Autodesk Inventor part; units mm, degrees
(part 2 of 2)
  line L759 (-171.45, -54.625) -> (-171.45, -57.15) construction
  line L760 (-164.45, -59.675) -> (-178.45, -59.675)
  line L761 (-178.45, -59.675) -> (-178.45, -60.275)
  line L762 (-178.45, -60.275) -> (-179.25, -60.275)
  line L763 (-179.25, -60.275) -> (-179.25, -73.075)
  line L764 (-179.25, -73.075) -> (-178.45, -73.075)
  line L765 (-178.45, -73.075) -> (-178.45, -73.675)
  line L766 (-178.45, -73.675) -> (-164.45, -73.675)
  line L767 (-164.45, -73.675) -> (-164.45, -73.075)
  line L768 (-164.45, -73.075) -> (-163.65, -73.075)
  line L769 (-163.65, -73.075) -> (-163.65, -60.275)
  line L770 (-163.65, -60.275) -> (-164.45, -60.275)
  line L771 (-164.45, -60.275) -> (-164.45, -59.675)
  line L772 (-161.925, -76.2) -> (-161.925, -57.15) construction
  line L773 (-161.925, -57.15) -> (-180.975, -57.15) construction
  line L774 (-180.975, -57.15) -> (-180.975, -76.2) construction
  line L775 (-180.975, -76.2) -> (-161.925, -76.2) construction
  line L776 (-161.925, -66.675) -> (-163.65, -66.675) construction
  line L777 (-179.25, -66.675) -> (-180.975, -66.675) construction
  line L778 (-171.45, -59.675) -> (-171.45, -57.15) construction
  line L779 (-171.45, -73.675) -> (-171.45, -76.2) construction
  line L780 (-164.45, -78.725) -> (-178.45, -78.725)
  line L781 (-178.45, -78.725) -> (-178.45, -79.325)
  line L782 (-178.45, -79.325) -> (-179.25, -79.325)
  line L783 (-179.25, -79.325) -> (-179.25, -92.125)
  line L784 (-179.25, -92.125) -> (-178.45, -92.125)
  line L785 (-178.45, -92.125) -> (-178.45, -92.725)
  line L786 (-178.45, -92.725) -> (-164.45, -92.725)
  line L787 (-164.45, -92.725) -> (-164.45, -92.125)
  line L788 (-164.45, -92.125) -> (-163.65, -92.125)
  line L789 (-163.65, -92.125) -> (-163.65, -79.325)
  line L790 (-163.65, -79.325) -> (-164.45, -79.325)
  line L791 (-164.45, -79.325) -> (-164.45, -78.725)
  line L792 (-161.925, -95.25) -> (-161.925, -76.2) construction
  line L793 (-161.925, -76.2) -> (-180.975, -76.2) construction
  line L794 (-180.975, -76.2) -> (-180.975, -95.25) construction
  line L795 (-180.975, -95.25) -> (-161.925, -95.25) construction
  line L796 (-161.925, -85.725) -> (-163.65, -85.725) construction
  line L797 (-179.25, -85.725) -> (-180.975, -85.725) construction
  line L798 (-171.45, -78.725) -> (-171.45, -76.2) construction
  line L799 (-171.45, -92.725) -> (-171.45, -95.25) construction
  line L800 (-183.5, -21.575) -> (-197.5, -21.575)
  line L801 (-197.5, -21.575) -> (-197.5, -22.175)
  line L802 (-197.5, -22.175) -> (-198.3, -22.175)
  line L803 (-198.3, -22.175) -> (-198.3, -34.975)
  line L804 (-198.3, -34.975) -> (-197.5, -34.975)
  line L805 (-197.5, -34.975) -> (-197.5, -35.575)
  line L806 (-197.5, -35.575) -> (-183.5, -35.575)
  line L807 (-183.5, -35.575) -> (-183.5, -34.975)
  line L808 (-183.5, -34.975) -> (-182.7, -34.975)
  line L809 (-182.7, -34.975) -> (-182.7, -22.175)
  line L810 (-182.7, -22.175) -> (-183.5, -22.175)
  line L811 (-183.5, -22.175) -> (-183.5, -21.575)
  line L812 (-180.975, -38.1) -> (-180.975, -19.05) construction
  line L813 (-180.975, -19.05) -> (-200.025, -19.05) construction
  line L814 (-200.025, -19.05) -> (-200.025, -38.1) construction
  line L815 (-200.025, -38.1) -> (-180.975, -38.1) construction
  line L816 (-180.975, -28.575) -> (-182.7, -28.575) construction
  line L817 (-198.3, -28.575) -> (-200.025, -28.575) construction
  line L818 (-190.5, -21.575) -> (-190.5, -19.05) construction
  line L819 (-190.5, -35.575) -> (-190.5, -38.1) construction
  line L820 (-183.5, -40.625) -> (-197.5, -40.625)
  line L821 (-197.5, -40.625) -> (-197.5, -41.225)
  line L822 (-197.5, -41.225) -> (-198.3, -41.225)
  line L823 (-198.3, -41.225) -> (-198.3, -54.025)
  line L824 (-198.3, -54.025) -> (-197.5, -54.025)
  line L825 (-197.5, -54.025) -> (-197.5, -54.625)
  line L826 (-197.5, -54.625) -> (-183.5, -54.625)
  line L827 (-183.5, -54.625) -> (-183.5, -54.025)
  line L828 (-183.5, -54.025) -> (-182.7, -54.025)
  line L829 (-182.7, -54.025) -> (-182.7, -41.225)
  line L830 (-182.7, -41.225) -> (-183.5, -41.225)
  line L831 (-183.5, -41.225) -> (-183.5, -40.625)
  line L832 (-180.975, -57.15) -> (-180.975, -38.1) construction
  line L833 (-180.975, -38.1) -> (-200.025, -38.1) construction
  line L834 (-200.025, -38.1) -> (-200.025, -57.15) construction
  line L835 (-200.025, -57.15) -> (-180.975, -57.15) construction
  line L836 (-180.975, -47.625) -> (-182.7, -47.625) construction
  line L837 (-198.3, -47.625) -> (-200.025, -47.625) construction
  line L838 (-190.5, -40.625) -> (-190.5, -38.1) construction
  line L839 (-190.5, -54.625) -> (-190.5, -57.15) construction
  line L840 (-183.5, -59.675) -> (-197.5, -59.675)
  line L841 (-197.5, -59.675) -> (-197.5, -60.275)
  line L842 (-197.5, -60.275) -> (-198.3, -60.275)
  line L843 (-198.3, -60.275) -> (-198.3, -73.075)
  line L844 (-198.3, -73.075) -> (-197.5, -73.075)
  line L845 (-197.5, -73.075) -> (-197.5, -73.675)
  line L846 (-197.5, -73.675) -> (-183.5, -73.675)
  line L847 (-183.5, -73.675) -> (-183.5, -73.075)
  line L848 (-183.5, -73.075) -> (-182.7, -73.075)
  line L849 (-182.7, -73.075) -> (-182.7, -60.275)
  line L850 (-182.7, -60.275) -> (-183.5, -60.275)
  line L851 (-183.5, -60.275) -> (-183.5, -59.675)
  line L852 (-180.975, -76.2) -> (-180.975, -57.15) construction
  line L853 (-180.975, -57.15) -> (-200.025, -57.15) construction
  line L854 (-200.025, -57.15) -> (-200.025, -76.2) construction
  line L855 (-200.025, -76.2) -> (-180.975, -76.2) construction
  line L856 (-180.975, -66.675) -> (-182.7, -66.675) construction
  line L857 (-198.3, -66.675) -> (-200.025, -66.675) construction
  line L858 (-190.5, -59.675) -> (-190.5, -57.15) construction
  line L859 (-190.5, -73.675) -> (-190.5, -76.2) construction
  line L860 (-183.5, -78.725) -> (-197.5, -78.725)
  line L861 (-197.5, -78.725) -> (-197.5, -79.325)
  line L862 (-197.5, -79.325) -> (-198.3, -79.325)
  line L863 (-198.3, -79.325) -> (-198.3, -92.125)
  line L864 (-198.3, -92.125) -> (-197.5, -92.125)
  line L865 (-197.5, -92.125) -> (-197.5, -92.725)
  line L866 (-197.5, -92.725) -> (-183.5, -92.725)
  line L867 (-183.5, -92.725) -> (-183.5, -92.125)
  line L868 (-183.5, -92.125) -> (-182.7, -92.125)
  line L869 (-182.7, -92.125) -> (-182.7, -79.325)
  line L870 (-182.7, -79.325) -> (-183.5, -79.325)
  line L871 (-183.5, -79.325) -> (-183.5, -78.725)
  line L872 (-180.975, -95.25) -> (-180.975, -76.2) construction
  line L873 (-180.975, -76.2) -> (-200.025, -76.2) construction
  line L874 (-200.025, -76.2) -> (-200.025, -95.25) construction
  line L875 (-200.025, -95.25) -> (-180.975, -95.25) construction
  line L876 (-180.975, -85.725) -> (-182.7, -85.725) construction
  line L877 (-198.3, -85.725) -> (-200.025, -85.725) construction
  line L878 (-190.5, -78.725) -> (-190.5, -76.2) construction
  line L879 (-190.5, -92.725) -> (-190.5, -95.25) construction
  line L880 (-202.55, -21.575) -> (-216.55, -21.575)
  line L881 (-216.55, -21.575) -> (-216.55, -22.175)
  line L882 (-216.55, -22.175) -> (-217.35, -22.175)
  line L883 (-217.35, -22.175) -> (-217.35, -34.975)
  line L884 (-217.35, -34.975) -> (-216.55, -34.975)
  line L885 (-216.55, -34.975) -> (-216.55, -35.575)
  line L886 (-216.55, -35.575) -> (-202.55, -35.575)
  line L887 (-202.55, -35.575) -> (-202.55, -34.975)
  line L888 (-202.55, -34.975) -> (-201.75, -34.975)
  line L889 (-201.75, -34.975) -> (-201.75, -22.175)
  line L890 (-201.75, -22.175) -> (-202.55, -22.175)
  line L891 (-202.55, -22.175) -> (-202.55, -21.575)
  line L892 (-200.025, -38.1) -> (-200.025, -19.05) construction
  line L893 (-200.025, -19.05) -> (-219.075, -19.05) construction
  line L894 (-219.075, -19.05) -> (-219.075, -38.1) construction
  line L895 (-219.075, -38.1) -> (-200.025, -38.1) construction
  line L896 (-200.025, -28.575) -> (-201.75, -28.575) construction
  line L897 (-217.35, -28.575) -> (-219.075, -28.575) construction
  line L898 (-209.55, -21.575) -> (-209.55, -19.05) construction
  line L899 (-209.55, -35.575) -> (-209.55, -38.1) construction
  line L900 (-202.55, -40.625) -> (-216.55, -40.625)
  line L901 (-216.55, -40.625) -> (-216.55, -41.225)
  line L902 (-216.55, -41.225) -> (-217.35, -41.225)
  line L903 (-217.35, -41.225) -> (-217.35, -54.025)
  line L904 (-217.35, -54.025) -> (-216.55, -54.025)
  line L905 (-216.55, -54.025) -> (-216.55, -54.625)
  line L906 (-216.55, -54.625) -> (-202.55, -54.625)
  line L907 (-202.55, -54.625) -> (-202.55, -54.025)
  line L908 (-202.55, -54.025) -> (-201.75, -54.025)
  line L909 (-201.75, -54.025) -> (-201.75, -41.225)
  line L910 (-201.75, -41.225) -> (-202.55, -41.225)
  line L911 (-202.55, -41.225) -> (-202.55, -40.625)
  line L912 (-200.025, -57.15) -> (-200.025, -38.1) construction
  line L913 (-200.025, -38.1) -> (-219.075, -38.1) construction
  line L914 (-219.075, -38.1) -> (-219.075, -57.15) construction
  line L915 (-219.075, -57.15) -> (-200.025, -57.15) construction
  line L916 (-200.025, -47.625) -> (-201.75, -47.625) construction
  line L917 (-217.35, -47.625) -> (-219.075, -47.625) construction
  line L918 (-209.55, -40.625) -> (-209.55, -38.1) construction
  line L919 (-209.55, -54.625) -> (-209.55, -57.15) construction
  line L920 (-202.55, -59.675) -> (-216.55, -59.675)
  line L921 (-216.55, -59.675) -> (-216.55, -60.275)
  line L922 (-216.55, -60.275) -> (-217.35, -60.275)
  line L923 (-217.35, -60.275) -> (-217.35, -73.075)
  line L924 (-217.35, -73.075) -> (-216.55, -73.075)
  line L925 (-216.55, -73.075) -> (-216.55, -73.675)
  line L926 (-216.55, -73.675) -> (-202.55, -73.675)
  line L927 (-202.55, -73.675) -> (-202.55, -73.075)
  line L928 (-202.55, -73.075) -> (-201.75, -73.075)
  line L929 (-201.75, -73.075) -> (-201.75, -60.275)
  line L930 (-201.75, -60.275) -> (-202.55, -60.275)
  line L931 (-202.55, -60.275) -> (-202.55, -59.675)
  line L932 (-200.025, -76.2) -> (-200.025, -57.15) construction
  line L933 (-200.025, -57.15) -> (-219.075, -57.15) construction
  line L934 (-219.075, -57.15) -> (-219.075, -76.2) construction
  line L935 (-219.075, -76.2) -> (-200.025, -76.2) construction
  line L936 (-200.025, -66.675) -> (-201.75, -66.675) construction
  line L937 (-217.35, -66.675) -> (-219.075, -66.675) construction
  line L938 (-209.55, -59.675) -> (-209.55, -57.15) construction
  line L939 (-209.55, -73.675) -> (-209.55, -76.2) construction
  line L940 (-202.55, -78.725) -> (-216.55, -78.725)
  line L941 (-216.55, -78.725) -> (-216.55, -79.325)
  line L942 (-216.55, -79.325) -> (-217.35, -79.325)
  line L943 (-217.35, -79.325) -> (-217.35, -92.125)
  line L944 (-217.35, -92.125) -> (-216.55, -92.125)
  line L945 (-216.55, -92.125) -> (-216.55, -92.725)
  line L946 (-216.55, -92.725) -> (-202.55, -92.725)
  line L947 (-202.55, -92.725) -> (-202.55, -92.125)
  line L948 (-202.55, -92.125) -> (-201.75, -92.125)
  line L949 (-201.75, -92.125) -> (-201.75, -79.325)
  line L950 (-201.75, -79.325) -> (-202.55, -79.325)
  line L951 (-202.55, -79.325) -> (-202.55, -78.725)
  line L952 (-200.025, -95.25) -> (-200.025, -76.2) construction
  line L953 (-200.025, -76.2) -> (-219.075, -76.2) construction
  line L954 (-219.075, -76.2) -> (-219.075, -95.25) construction
  line L955 (-219.075, -95.25) -> (-200.025, -95.25) construction
  line L956 (-200.025, -85.725) -> (-201.75, -85.725) construction
  line L957 (-217.35, -85.725) -> (-219.075, -85.725) construction
  line L958 (-209.55, -78.725) -> (-209.55, -76.2) construction
  line L959 (-209.55, -92.725) -> (-209.55, -95.25) construction
  line L960 (-221.6, -21.575) -> (-235.6, -21.575)
  line L961 (-235.6, -21.575) -> (-235.6, -22.175)
  line L962 (-235.6, -22.175) -> (-236.4, -22.175)
  line L963 (-236.4, -22.175) -> (-236.4, -34.975)
  line L964 (-236.4, -34.975) -> (-235.6, -34.975)
  line L965 (-235.6, -34.975) -> (-235.6, -35.575)
  line L966 (-235.6, -35.575) -> (-221.6, -35.575)
  line L967 (-221.6, -35.575) -> (-221.6, -34.975)
  line L968 (-221.6, -34.975) -> (-220.8, -34.975)
  line L969 (-220.8, -34.975) -> (-220.8, -22.175)
  line L970 (-220.8, -22.175) -> (-221.6, -22.175)
  line L971 (-221.6, -22.175) -> (-221.6, -21.575)
  line L972 (-219.075, -38.1) -> (-219.075, -19.05) construction
  line L973 (-219.075, -19.05) -> (-238.125, -19.05) construction
  line L974 (-238.125, -19.05) -> (-238.125, -38.1) construction
  line L975 (-238.125, -38.1) -> (-219.075, -38.1) construction
  line L976 (-219.075, -28.575) -> (-220.8, -28.575) construction
  line L977 (-236.4, -28.575) -> (-238.125, -28.575) construction
  line L978 (-228.6, -21.575) -> (-228.6, -19.05) construction
  line L979 (-228.6, -35.575) -> (-228.6, -38.1) construction
  line L980 (-221.6, -40.625) -> (-235.6, -40.625)
  line L981 (-235.6, -40.625) -> (-235.6, -41.225)
  line L982 (-235.6, -41.225) -> (-236.4, -41.225)
  line L983 (-236.4, -41.225) -> (-236.4, -54.025)
  line L984 (-236.4, -54.025) -> (-235.6, -54.025)
  line L985 (-235.6, -54.025) -> (-235.6, -54.625)
  line L986 (-235.6, -54.625) -> (-221.6, -54.625)
  line L987 (-221.6, -54.625) -> (-221.6, -54.025)
  line L988 (-221.6, -54.025) -> (-220.8, -54.025)
  line L989 (-220.8, -54.025) -> (-220.8, -41.225)
  line L990 (-220.8, -41.225) -> (-221.6, -41.225)
  line L991 (-221.6, -41.225) -> (-221.6, -40.625)
  line L992 (-219.075, -57.15) -> (-219.075, -38.1) construction
  line L993 (-219.075, -38.1) -> (-238.125, -38.1) construction
  line L994 (-238.125, -38.1) -> (-238.125, -57.15) construction
  line L995 (-238.125, -57.15) -> (-219.075, -57.15) construction
  line L996 (-219.075, -47.625) -> (-220.8, -47.625) construction
  line L997 (-236.4, -47.625) -> (-238.125, -47.625) construction
  line L998 (-228.6, -40.625) -> (-228.6, -38.1) construction
  line L999 (-228.6, -54.625) -> (-228.6, -57.15) construction
  line L1000 (-221.6, -59.675) -> (-235.6, -59.675)
  line L1001 (-235.6, -59.675) -> (-235.6, -60.275)
  line L1002 (-235.6, -60.275) -> (-236.4, -60.275)
  line L1003 (-236.4, -60.275) -> (-236.4, -73.075)
  line L1004 (-236.4, -73.075) -> (-235.6, -73.075)
  line L1005 (-235.6, -73.075) -> (-235.6, -73.675)
  line L1006 (-235.6, -73.675) -> (-221.6, -73.675)
  line L1007 (-221.6, -73.675) -> (-221.6, -73.075)
  line L1008 (-221.6, -73.075) -> (-220.8, -73.075)
  line L1009 (-220.8, -73.075) -> (-220.8, -60.275)
  line L1010 (-220.8, -60.275) -> (-221.6, -60.275)
  line L1011 (-221.6, -60.275) -> (-221.6, -59.675)
  line L1012 (-219.075, -76.2) -> (-219.075, -57.15) construction
  line L1013 (-219.075, -57.15) -> (-238.125, -57.15) construction
  line L1014 (-238.125, -57.15) -> (-238.125, -76.2) construction
  line L1015 (-238.125, -76.2) -> (-219.075, -76.2) construction
  line L1016 (-219.075, -66.675) -> (-220.8, -66.675) construction
  line L1017 (-236.4, -66.675) -> (-238.125, -66.675) construction
  line L1018 (-228.6, -59.675) -> (-228.6, -57.15) construction
  line L1019 (-228.6, -73.675) -> (-228.6, -76.2) construction
  line L1020 (-221.6, -78.725) -> (-235.6, -78.725)
  line L1021 (-235.6, -78.725) -> (-235.6, -79.325)
  line L1022 (-235.6, -79.325) -> (-236.4, -79.325)
  line L1023 (-236.4, -79.325) -> (-236.4, -92.125)
  line L1024 (-236.4, -92.125) -> (-235.6, -92.125)
  line L1025 (-235.6, -92.125) -> (-235.6, -92.725)
  line L1026 (-235.6, -92.725) -> (-221.6, -92.725)
  line L1027 (-221.6, -92.725) -> (-221.6, -92.125)
  line L1028 (-221.6, -92.125) -> (-220.8, -92.125)
  line L1029 (-220.8, -92.125) -> (-220.8, -79.325)
  line L1030 (-220.8, -79.325) -> (-221.6, -79.325)
  line L1031 (-221.6, -79.325) -> (-221.6, -78.725)
  line L1032 (-219.075, -95.25) -> (-219.075, -76.2) construction
  line L1033 (-219.075, -76.2) -> (-238.125, -76.2) construction
  line L1034 (-238.125, -76.2) -> (-238.125, -95.25) construction
  line L1035 (-238.125, -95.25) -> (-219.075, -95.25) construction
  line L1036 (-219.075, -85.725) -> (-220.8, -85.725) construction
  line L1037 (-236.4, -85.725) -> (-238.125, -85.725) construction
  line L1038 (-228.6, -78.725) -> (-228.6, -76.2) construction
  line L1039 (-228.6, -92.725) -> (-228.6, -95.25) construction
  line L1040 (-240.65, -21.575) -> (-254.65, -21.575)
  line L1041 (-254.65, -21.575) -> (-254.65, -22.175)
  line L1042 (-254.65, -22.175) -> (-255.45, -22.175)
  line L1043 (-255.45, -22.175) -> (-255.45, -34.975)
  line L1044 (-255.45, -34.975) -> (-254.65, -34.975)
  line L1045 (-254.65, -34.975) -> (-254.65, -35.575)
  line L1046 (-254.65, -35.575) -> (-240.65, -35.575)
  line L1047 (-240.65, -35.575) -> (-240.65, -34.975)
  line L1048 (-240.65, -34.975) -> (-239.85, -34.975)
  line L1049 (-239.85, -34.975) -> (-239.85, -22.175)
  line L1050 (-239.85, -22.175) -> (-240.65, -22.175)
  line L1051 (-240.65, -22.175) -> (-240.65, -21.575)
  line L1052 (-238.125, -38.1) -> (-238.125, -19.05) construction
  line L1053 (-238.125, -19.05) -> (-257.175, -19.05) construction
  line L1054 (-257.175, -19.05) -> (-257.175, -38.1) construction
  line L1055 (-257.175, -38.1) -> (-238.125, -38.1) construction
  line L1056 (-238.125, -28.575) -> (-239.85, -28.575) construction
  line L1057 (-255.45, -28.575) -> (-257.175, -28.575) construction
  line L1058 (-247.65, -21.575) -> (-247.65, -19.05) construction
  line L1059 (-247.65, -35.575) -> (-247.65, -38.1) construction
  line L1060 (-240.65, -40.625) -> (-254.65, -40.625)
  line L1061 (-254.65, -40.625) -> (-254.65, -41.225)
  line L1062 (-254.65, -41.225) -> (-255.45, -41.225)
  line L1063 (-255.45, -41.225) -> (-255.45, -54.025)
  line L1064 (-255.45, -54.025) -> (-254.65, -54.025)
  line L1065 (-254.65, -54.025) -> (-254.65, -54.625)
  line L1066 (-254.65, -54.625) -> (-240.65, -54.625)
  line L1067 (-240.65, -54.625) -> (-240.65, -54.025)
  line L1068 (-240.65, -54.025) -> (-239.85, -54.025)
  line L1069 (-239.85, -54.025) -> (-239.85, -41.225)
  line L1070 (-239.85, -41.225) -> (-240.65, -41.225)
  line L1071 (-240.65, -41.225) -> (-240.65, -40.625)
  line L1072 (-238.125, -57.15) -> (-238.125, -38.1) construction
  line L1073 (-238.125, -38.1) -> (-257.175, -38.1) construction
  line L1074 (-257.175, -38.1) -> (-257.175, -57.15) construction
  line L1075 (-257.175, -57.15) -> (-238.125, -57.15) construction
  line L1076 (-238.125, -47.625) -> (-239.85, -47.625) construction
  line L1077 (-255.45, -47.625) -> (-257.175, -47.625) construction
  line L1078 (-247.65, -40.625) -> (-247.65, -38.1) construction
  line L1079 (-247.65, -54.625) -> (-247.65, -57.15) construction
  line L1080 (-240.65, -59.675) -> (-254.65, -59.675)
  line L1081 (-254.65, -59.675) -> (-254.65, -60.275)
  line L1082 (-254.65, -60.275) -> (-255.45, -60.275)
  line L1083 (-255.45, -60.275) -> (-255.45, -73.075)
  line L1084 (-255.45, -73.075) -> (-254.65, -73.075)
  line L1085 (-254.65, -73.075) -> (-254.65, -73.675)
  line L1086 (-254.65, -73.675) -> (-240.65, -73.675)
  line L1087 (-240.65, -73.675) -> (-240.65, -73.075)
  line L1088 (-240.65, -73.075) -> (-239.85, -73.075)
  line L1089 (-239.85, -73.075) -> (-239.85, -60.275)
  line L1090 (-239.85, -60.275) -> (-240.65, -60.275)
  line L1091 (-240.65, -60.275) -> (-240.65, -59.675)
  line L1092 (-238.125, -76.2) -> (-238.125, -57.15) construction
  line L1093 (-238.125, -57.15) -> (-257.175, -57.15) construction
  line L1094 (-257.175, -57.15) -> (-257.175, -76.2) construction
  line L1095 (-257.175, -76.2) -> (-238.125, -76.2) construction
  line L1096 (-238.125, -66.675) -> (-239.85, -66.675) construction
  line L1097 (-255.45, -66.675) -> (-257.175, -66.675) construction
  line L1098 (-247.65, -59.675) -> (-247.65, -57.15) construction
  line L1099 (-247.65, -73.675) -> (-247.65, -76.2) construction
  line L1100 (-240.65, -78.725) -> (-254.65, -78.725)
  line L1101 (-254.65, -78.725) -> (-254.65, -79.325)
  line L1102 (-254.65, -79.325) -> (-255.45, -79.325)
  line L1103 (-255.45, -79.325) -> (-255.45, -92.125)
  line L1104 (-255.45, -92.125) -> (-254.65, -92.125)
  line L1105 (-254.65, -92.125) -> (-254.65, -92.725)
  line L1106 (-254.65, -92.725) -> (-240.65, -92.725)
  line L1107 (-240.65, -92.725) -> (-240.65, -92.125)
  line L1108 (-240.65, -92.125) -> (-239.85, -92.125)
  line L1109 (-239.85, -92.125) -> (-239.85, -79.325)
  line L1110 (-239.85, -79.325) -> (-240.65, -79.325)
  line L1111 (-240.65, -79.325) -> (-240.65, -78.725)
  line L1112 (-238.125, -95.25) -> (-238.125, -76.2) construction
  line L1113 (-238.125, -76.2) -> (-257.175, -76.2) construction
  line L1114 (-257.175, -76.2) -> (-257.175, -95.25) construction
  line L1115 (-257.175, -95.25) -> (-238.125, -95.25) construction
  line L1116 (-238.125, -85.725) -> (-239.85, -85.725) construction
  line L1117 (-255.45, -85.725) -> (-257.175, -85.725) construction
  line L1118 (-247.65, -78.725) -> (-247.65, -76.2) construction
  line L1119 (-247.65, -92.725) -> (-247.65, -95.25) construction
  line L1120 (-266.8438, -2.525) -> (-280.8438, -2.525)
  line L1121 (-280.8438, -2.525) -> (-280.8438, -3.125)
  line L1122 (-280.8438, -3.125) -> (-281.6438, -3.125)
  line L1123 (-281.6438, -3.125) -> (-281.6438, -15.925)
  line L1124 (-281.6438, -15.925) -> (-280.8438, -15.925)
  line L1125 (-280.8438, -15.925) -> (-280.8438, -16.525)
  line L1126 (-280.8438, -16.525) -> (-266.8438, -16.525)
  line L1127 (-266.8438, -16.525) -> (-266.8438, -15.925)
  line L1128 (-266.8438, -15.925) -> (-266.0438, -15.925)
  line L1129 (-266.0438, -15.925) -> (-266.0438, -3.125)
  line L1130 (-266.0438, -3.125) -> (-266.8438, -3.125)
  line L1131 (-266.8438, -3.125) -> (-266.8438, -2.525)
  line L1132 (-261.9375, -19.05) -> (-261.9375, 0) construction
  line L1133 (-261.9375, 0) -> (-285.75, 0) construction
  line L1134 (-285.75, 0) -> (-285.75, -19.05) construction
  line L1135 (-285.75, -19.05) -> (-261.9375, -19.05) construction
  line L1136 (-261.9375, -9.525) -> (-266.0438, -9.525) construction
  line L1137 (-281.6438, -9.525) -> (-285.75, -9.525) construction
  line L1138 (-273.8438, -2.525) -> (-273.8438, 0) construction
  line L1139 (-273.8438, -16.525) -> (-273.8438, -19.05) construction
  line L1140 (-243.0312, -2.525) -> (-257.0313, -2.525)
  line L1141 (-257.0313, -2.525) -> (-257.0312, -3.125)
  line L1142 (-257.0312, -3.125) -> (-257.8313, -3.125)
  line L1143 (-257.8313, -3.125) -> (-257.8313, -15.925)
  line L1144 (-257.8313, -15.925) -> (-257.0312, -15.925)
  line L1145 (-257.0312, -15.925) -> (-257.0313, -16.525)
  line L1146 (-257.0313, -16.525) -> (-243.0312, -16.525)
  line L1147 (-243.0312, -16.525) -> (-243.0313, -15.925)
  line L1148 (-243.0313, -15.925) -> (-242.2313, -15.925)
  line L1149 (-242.2313, -15.925) -> (-242.2313, -3.125)
  line L1150 (-242.2313, -3.125) -> (-243.0313, -3.125)
  line L1151 (-243.0313, -3.125) -> (-243.0312, -2.525)
  line L1152 (-238.125, -19.05) -> (-238.125, 0) construction
  line L1153 (-238.125, 0) -> (-261.9375, 0) construction
  line L1154 (-261.9375, 0) -> (-261.9375, -19.05) construction
  line L1155 (-261.9375, -19.05) -> (-238.125, -19.05) construction
  line L1156 (-238.125, -9.525) -> (-242.2313, -9.525) construction
  line L1157 (-257.8312, -9.525) -> (-261.9375, -9.525) construction
  line L1158 (-250.0313, -2.525) -> (-250.0313, 0) construction
  line L1159 (-250.0313, -16.525) -> (-250.0313, -19.05) construction
  line L1160 (-219.2188, -2.525) -> (-233.2188, -2.525)
  line L1161 (-233.2188, -2.525) -> (-233.2188, -3.125)
  line L1162 (-233.2188, -3.125) -> (-234.0188, -3.125)
  line L1163 (-234.0188, -3.125) -> (-234.0188, -15.925)
  line L1164 (-234.0188, -15.925) -> (-233.2188, -15.925)
  line L1165 (-233.2188, -15.925) -> (-233.2188, -16.525)
  line L1166 (-233.2188, -16.525) -> (-219.2188, -16.525)
  line L1167 (-219.2188, -16.525) -> (-219.2188, -15.925)
  line L1168 (-219.2188, -15.925) -> (-218.4188, -15.925)
  line L1169 (-218.4188, -15.925) -> (-218.4188, -3.125)
  line L1170 (-218.4188, -3.125) -> (-219.2188, -3.125)
  line L1171 (-219.2188, -3.125) -> (-219.2188, -2.525)
  line L1172 (-214.3125, -19.05) -> (-214.3125, 0) construction
  line L1173 (-214.3125, 0) -> (-238.125, 0) construction
  line L1174 (-238.125, 0) -> (-238.125, -19.05) construction
  line L1175 (-238.125, -19.05) -> (-214.3125, -19.05) construction
  line L1176 (-214.3125, -9.525) -> (-218.4188, -9.525) construction
  line L1177 (-234.0187, -9.525) -> (-238.125, -9.525) construction
  line L1178 (-226.2188, -2.525) -> (-226.2188, 0) construction
  line L1179 (-226.2188, -16.525) -> (-226.2188, -19.05) construction
  line L1180 (-195.4062, -2.525) -> (-209.4062, -2.525)
  line L1181 (-209.4062, -2.525) -> (-209.4062, -3.125)
  line L1182 (-209.4062, -3.125) -> (-210.2062, -3.125)
  line L1183 (-210.2062, -3.125) -> (-210.2062, -15.925)
  line L1184 (-210.2062, -15.925) -> (-209.4062, -15.925)
  line L1185 (-209.4062, -15.925) -> (-209.4062, -16.525)
  line L1186 (-209.4062, -16.525) -> (-195.4062, -16.525)
  line L1187 (-195.4062, -16.525) -> (-195.4063, -15.925)
  line L1188 (-195.4063, -15.925) -> (-194.6062, -15.925)
  line L1189 (-194.6062, -15.925) -> (-194.6062, -3.125)
  line L1190 (-194.6062, -3.125) -> (-195.4063, -3.125)
  line L1191 (-195.4063, -3.125) -> (-195.4062, -2.525)
  line L1192 (-190.5, -19.05) -> (-190.5, 0) construction
  line L1193 (-190.5, 0) -> (-214.3125, 0) construction
  line L1194 (-214.3125, 0) -> (-214.3125, -19.05) construction
  line L1195 (-214.3125, -19.05) -> (-190.5, -19.05) construction
  line L1196 (-190.5, -9.525) -> (-194.6063, -9.525) construction
  line L1197 (-210.2062, -9.525) -> (-214.3125, -9.525) construction
  line L1198 (-202.4062, -2.525) -> (-202.4062, 0) construction
  line L1199 (-202.4062, -16.525) -> (-202.4062, -19.05) construction
  line L1200 (-264.4625, -21.575) -> (-278.4625, -21.575)
  line L1201 (-278.4625, -21.575) -> (-278.4625, -22.175)
  line L1202 (-278.4625, -22.175) -> (-279.2625, -22.175)
  line L1203 (-279.2625, -22.175) -> (-279.2625, -34.975)
  line L1204 (-279.2625, -34.975) -> (-278.4625, -34.975)
  line L1205 (-278.4625, -34.975) -> (-278.4625, -35.575)
  line L1206 (-278.4625, -35.575) -> (-264.4625, -35.575)
  line L1207 (-264.4625, -35.575) -> (-264.4625, -34.975)
  line L1208 (-264.4625, -34.975) -> (-263.6625, -34.975)
  line L1209 (-263.6625, -34.975) -> (-263.6625, -22.175)
  line L1210 (-263.6625, -22.175) -> (-264.4625, -22.175)
  line L1211 (-264.4625, -22.175) -> (-264.4625, -21.575)
  line L1212 (-257.175, -38.1) -> (-257.175, -19.05) construction
  line L1213 (-257.175, -19.05) -> (-285.75, -19.05) construction
  line L1214 (-285.75, -19.05) -> (-285.75, -38.1) construction
  line L1215 (-285.75, -38.1) -> (-257.175, -38.1) construction
  line L1216 (-257.175, -28.575) -> (-263.6625, -28.575) construction
  line L1217 (-279.2625, -28.575) -> (-285.75, -28.575) construction
  line L1218 (-271.4625, -21.575) -> (-271.4625, -19.05) construction
  line L1219 (-271.4625, -35.575) -> (-271.4625, -38.1) construction
  line L1220 (-264.4625, -40.625) -> (-278.4625, -40.625)
  line L1221 (-278.4625, -40.625) -> (-278.4625, -41.225)
  line L1222 (-278.4625, -41.225) -> (-279.2625, -41.225)
  line L1223 (-279.2625, -41.225) -> (-279.2625, -54.025)
  line L1224 (-279.2625, -54.025) -> (-278.4625, -54.025)
  line L1225 (-278.4625, -54.025) -> (-278.4625, -54.625)
  line L1226 (-278.4625, -54.625) -> (-264.4625, -54.625)
  line L1227 (-264.4625, -54.625) -> (-264.4625, -54.025)
  line L1228 (-264.4625, -54.025) -> (-263.6625, -54.025)
  line L1229 (-263.6625, -54.025) -> (-263.6625, -41.225)
  line L1230 (-263.6625, -41.225) -> (-264.4625, -41.225)
  line L1231 (-264.4625, -41.225) -> (-264.4625, -40.625)
  line L1232 (-257.175, -57.15) -> (-257.175, -38.1) construction
  line L1233 (-257.175, -38.1) -> (-285.75, -38.1) construction
  line L1234 (-285.75, -38.1) -> (-285.75, -57.15) construction
  line L1235 (-285.75, -57.15) -> (-257.175, -57.15) construction
  line L1236 (-257.175, -47.625) -> (-263.6625, -47.625) construction
  line L1237 (-279.2625, -47.625) -> (-285.75, -47.625) construction
  line L1238 (-271.4625, -40.625) -> (-271.4625, -38.1) construction
  line L1239 (-271.4625, -54.625) -> (-271.4625, -57.15) construction
  line L1240 (-264.4625, -59.675) -> (-278.4625, -59.675)
  line L1241 (-278.4625, -59.675) -> (-278.4625, -60.275)
  line L1242 (-278.4625, -60.275) -> (-279.2625, -60.275)
  line L1243 (-279.2625, -60.275) -> (-279.2625, -73.075)
  line L1244 (-279.2625, -73.075) -> (-278.4625, -73.075)
  line L1245 (-278.4625, -73.075) -> (-278.4625, -73.675)
  line L1246 (-278.4625, -73.675) -> (-264.4625, -73.675)
  line L1247 (-264.4625, -73.675) -> (-264.4625, -73.075)
  line L1248 (-264.4625, -73.075) -> (-263.6625, -73.075)
  line L1249 (-263.6625, -73.075) -> (-263.6625, -60.275)
  line L1250 (-263.6625, -60.275) -> (-264.4625, -60.275)
  line L1251 (-264.4625, -60.275) -> (-264.4625, -59.675)
  line L1252 (-257.175, -76.2) -> (-257.175, -57.15) construction
  line L1253 (-257.175, -57.15) -> (-285.75, -57.15) construction
  line L1254 (-285.75, -57.15) -> (-285.75, -76.2) construction
  line L1255 (-285.75, -76.2) -> (-257.175, -76.2) construction
  line L1256 (-257.175, -66.675) -> (-263.6625, -66.675) construction
  line L1257 (-279.2625, -66.675) -> (-285.75, -66.675) construction
  line L1258 (-271.4625, -59.675) -> (-271.4625, -57.15) construction
  line L1259 (-271.4625, -73.675) -> (-271.4625, -76.2) construction
  line L1260 (-264.4625, -78.725) -> (-278.4625, -78.725)
  line L1261 (-278.4625, -78.725) -> (-278.4625, -79.325)
  line L1262 (-278.4625, -79.325) -> (-279.2625, -79.325)
  line L1263 (-279.2625, -79.325) -> (-279.2625, -92.125)
  line L1264 (-279.2625, -92.125) -> (-278.4625, -92.125)
  line L1265 (-278.4625, -92.125) -> (-278.4625, -92.725)
  line L1266 (-278.4625, -92.725) -> (-264.4625, -92.725)
  line L1267 (-264.4625, -92.725) -> (-264.4625, -92.125)
  line L1268 (-264.4625, -92.125) -> (-263.6625, -92.125)
  line L1269 (-263.6625, -92.125) -> (-263.6625, -79.325)
  line L1270 (-263.6625, -79.325) -> (-264.4625, -79.325)
  line L1271 (-264.4625, -79.325) -> (-264.4625, -78.725)
  line L1272 (-257.175, -95.25) -> (-257.175, -76.2) construction
  line L1273 (-257.175, -76.2) -> (-285.75, -76.2) construction
  line L1274 (-285.75, -76.2) -> (-285.75, -95.25) construction
  line L1275 (-285.75, -95.25) -> (-257.175, -95.25) construction
  line L1276 (-257.175, -85.725) -> (-263.6625, -85.725) construction
  line L1277 (-279.2625, -85.725) -> (-285.75, -85.725) construction
  line L1278 (-271.4625, -78.725) -> (-271.4625, -76.2) construction
  line L1279 (-271.4625, -92.725) -> (-271.4625, -95.25) construction
  line L1280 (-169.2125, -2.525) -> (-183.2125, -2.525)
  line L1281 (-183.2125, -2.525) -> (-183.2125, -3.125)
  line L1282 (-183.2125, -3.125) -> (-184.0125, -3.125)
  line L1283 (-184.0125, -3.125) -> (-184.0125, -15.925)
  line L1284 (-184.0125, -15.925) -> (-183.2125, -15.925)
  line L1285 (-183.2125, -15.925) -> (-183.2125, -16.525)
  line L1286 (-183.2125, -16.525) -> (-169.2125, -16.525)
  line L1287 (-169.2125, -16.525) -> (-169.2125, -15.925)
  line L1288 (-169.2125, -15.925) -> (-168.4125, -15.925)
  line L1289 (-168.4125, -15.925) -> (-168.4125, -3.125)
  line L1290 (-168.4125, -3.125) -> (-169.2125, -3.125)
  line L1291 (-169.2125, -3.125) -> (-169.2125, -2.525)
  line L1292 (-161.925, -19.05) -> (-161.925, 0) construction
  line L1293 (-161.925, 0) -> (-190.5, 0) construction
  line L1294 (-190.5, 0) -> (-190.5, -19.05) construction
  line L1295 (-190.5, -19.05) -> (-161.925, -19.05) construction
  line L1296 (-161.925, -9.525) -> (-168.4125, -9.525) construction
  line L1297 (-184.0125, -9.525) -> (-190.5, -9.525) construction
  line L1298 (-176.2125, -2.525) -> (-176.2125, 0) construction
  line L1299 (-176.2125, -16.525) -> (-176.2125, -19.05) construction
  line L1300 (-102.5375, -2.525) -> (-116.5375, -2.525)
  line L1301 (-116.5375, -2.525) -> (-116.5375, -3.125)
  line L1302 (-116.5375, -3.125) -> (-117.3375, -3.125)
  line L1303 (-117.3375, -3.125) -> (-117.3375, -15.925)
  line L1304 (-117.3375, -15.925) -> (-116.5375, -15.925)
  line L1305 (-116.5375, -15.925) -> (-116.5375, -16.525)
  line L1306 (-116.5375, -16.525) -> (-102.5375, -16.525)
  line L1307 (-102.5375, -16.525) -> (-102.5375, -15.925)
  line L1308 (-102.5375, -15.925) -> (-101.7375, -15.925)
  line L1309 (-101.7375, -15.925) -> (-101.7375, -3.125)
  line L1310 (-101.7375, -3.125) -> (-102.5375, -3.125)
  line L1311 (-102.5375, -3.125) -> (-102.5375, -2.525)
  line L1312 (-95.25, -19.05) -> (-95.25, 0) construction
  line L1313 (-95.25, 0) -> (-123.825, 0) construction
  line L1314 (-123.825, 0) -> (-123.825, -19.05) construction
  line L1315 (-123.825, -19.05) -> (-95.25, -19.05) construction
  line L1316 (-95.25, -9.525) -> (-101.7375, -9.525) construction
  line L1317 (-117.3375, -9.525) -> (-123.825, -9.525) construction
  line L1318 (-109.5375, -2.525) -> (-109.5375, 0) construction
  line L1319 (-109.5375, -16.525) -> (-109.5375, -19.05) construction
  line L1320 (-123.825, -9.525) -> (-135.075, -9.525) construction
  line L1321 (-135.075, -15.925) -> (-135.075, -3.125)
  line L1322 (-123.825, -19.05) -> (-123.825, 0) construction
  line L1323 (-135.875, -15.925) -> (-135.075, -15.925)
  line L1324 (-135.875, -16.525) -> (-135.875, -15.925)
  line L1325 (-161.925, -19.05) -> (-123.825, -19.05) construction
  line L1326 (-123.825, 0) -> (-161.925, 0) construction
  line L1327 (-142.875, -2.525) -> (-142.875, 0) construction
  line L1328 (-142.875, -16.525) -> (-142.875, -19.05) construction
  line L1329 (-149.875, -16.525) -> (-135.875, -16.525)
  line L1330 (-135.875, -2.525) -> (-149.875, -2.525)
  line L1331 (-149.875, -15.925) -> (-149.875, -16.525)
  line L1332 (-150.675, -15.925) -> (-149.875, -15.925)
  line L1333 (-150.675, -3.125) -> (-150.675, -15.925)
  line L1334 (-149.875, -2.525) -> (-149.875, -3.125)
  line L1335 (-149.875, -3.125) -> (-150.675, -3.125)
  line L1336 (-158.475, -1.765) -> (-155.275, -1.765)
  line L1337 (-135.875, -3.125) -> (-135.875, -2.525)
  line L1338 (-135.075, -3.125) -> (-135.875, -3.125)
  line L1339 (-127.275, -1.765) -> (-130.475, -1.765)
  line L1340 (-130.475, -1.765) -> (-130.475, -15.765)
  line L1341 (-128.875, -15.765) -> (-128.875, -1.765) construction
  line L1342 (-127.275, -15.765) -> (-127.275, -1.765)
  line L1343 (-127.275, -8.765) -> (-130.475, -8.765) construction
  line L1344 (-130.475, -15.765) -> (-127.275, -15.765)
  line L1345 (-158.475, -8.765) -> (-155.275, -8.765) construction
  line L1346 (-155.275, -1.765) -> (-155.275, -15.765)
  line L1347 (-150.675, -9.525) -> (-161.925, -9.525) construction
  line L1348 (-156.875, -15.765) -> (-156.875, -1.765) construction
  line L1349 (-158.475, -15.765) -> (-158.475, -1.765)
  line L1350 (-161.925, 0) -> (-161.925, -19.05) construction
  line L1351 (-155.275, -15.765) -> (-158.475, -15.765)
  line L1352 (0, 0) -> (-285.75, 0)
  line L1353 (-285.75, 0) -> (-285.75, -95.25)
  line L1354 (-285.75, -95.25) -> (0, -95.25)
  line L1355 (0, -95.25) -> (0, 0)
  dimension "d199" = 12.8
  dimension "d200" = 14
  dimension "d201" = 14
  dimension "d202" = 15.6
  dimension "d203" = 23.8125
  dimension "d204" = 19.05
  dimension "d208" = 23.8125
  dimension "d213" = 12.8
  dimension "d214" = 14
  dimension "d215" = 14
  dimension "d216" = 15.6
  dimension "d217" = 28.575
  dimension "d218" = 19.05
  dimension "d222" = 19.05
  dimension "d227" = 12.8
  dimension "d228" = 14
  dimension "d229" = 14
  dimension "d230" = 15.6
  dimension "d231" = 19.05
  dimension "d232" = 19.05
  dimension "d235" = 19.05
  dimension "d238" = 19.05
  dimension "d241" = 12.8
  dimension "d242" = 14
  dimension "d243" = 14
  dimension "d244" = 15.6
  dimension "d245" = 23.8125
  dimension "d246" = 19.05
  dimension "d250" = 23.8125
  dimension "d255" = 12.8
  dimension "d256" = 14
  dimension "d257" = 14
  dimension "d258" = 15.6
  dimension "d259" = 28.575
  dimension "d260" = 19.05
  dimension "d264" = 19.05
  dimension "d269" = 12.8
  dimension "d270" = 14
  dimension "d271" = 14
  dimension "d272" = 15.6
  dimension "d273" = 28.575
  dimension "d274" = 19.05
  dimension "d276" = 12.8
  dimension "d277" = 14
  dimension "d278" = 14
  dimension "d279" = 15.6
  dimension "d280" = 28.575
  dimension "d281" = 19.05
  dimension "d283" = 12.8
  dimension "d284" = 14
  dimension "d285" = 14
  dimension "d286" = 15.6
  dimension "d287" = 38.1
  dimension "d288" = 19.05
  dimension "d289" = 3.2
  dimension "d290" = 14
  dimension "d291" = 14
  dimension "d292" = 0.76
  dimension "d294" = 285.75
  dimension "d295" = 95.25
  constraints: 2712 end point, 469 point on line, 116 perpendicular, 68 midpoint, 54 collinear, 12 horizontal, 12 vertical, 10 parallel, 8 symmetric about line, 7 coincident, 2590 other
  measures "d199" distance of L8.end L9.end
  measures "d200" distance between parallel lines of L0 L6
  measures "d201" distance of L5.end L6.end
  measures "d202" distance between parallel lines of L3 L9
  measures "d203" distance of L14.end L12.start
  measures "d204" distance of L12.start L12.end
  measures "d208" distance of L16.start L36.start
  measures "d213" distance of L88.end L89.end
  measures "d214" distance between parallel lines of L80 L86
  measures "d215" distance of L85.end L86.end
  measures "d216" distance between parallel lines of L83 L89
  measures "d217" distance of L94.end L92.start
  measures "d218" distance of L92.start L92.end
  measures "d222" distance of L97.start L117.start
  measures "d227" distance of L168.end L169.end
  measures "d228" distance between parallel lines of L160 L166
  measures "d229" distance of L165.end L166.end
  measures "d230" distance between parallel lines of L163 L169
  measures "d231" distance of L174.end L172.start
  measures "d232" distance of L172.start L172.end
  measures "d235" distance of L178.start L198.start
  measures "d238" distance of L178.start L258.start
  measures "d241" distance of L1128.end L1129.end
  measures "d242" distance between parallel lines of L1120 L1126
  measures "d243" distance of L1125.end L1126.end
  measures "d244" distance between parallel lines of L1123 L1129
  measures "d245" distance of L1134.end L1132.start
  measures "d246" distance of L1132.start L1132.end
  measures "d250" distance of L1125.end L1145.end
  measures "d255" distance of L1208.end L1209.end
  measures "d256" distance between parallel lines of L1200 L1206
  measures "d257" distance of L1205.end L1206.end
  measures "d258" distance between parallel lines of L1203 L1209
  measures "d259" distance of L1214.end L1212.start
  measures "d260" distance of L1212.start L1212.end
  measures "d264" distance of L1213.end L1234.start
  measures "d269" distance of L1288.end L1289.end
  measures "d270" distance between parallel lines of L1280 L1286
  measures "d271" distance of L1285.end L1286.end
  measures "d272" distance between parallel lines of L1283 L1289
  measures "d273" distance of L1294.end L1292.start
  measures "d274" distance of L1292.start L1292.end
  measures "d276" distance of L1308.end L1309.end
  measures "d277" distance between parallel lines of L1300 L1306
  measures "d278" distance of L1305.end L1306.end
  measures "d279" distance between parallel lines of L1303 L1309
  measures "d280" distance of L1314.end L1312.start
  measures "d281" distance of L1312.start L1312.end
  measures "d283" distance of L1321.start L1321.end
  measures "d284" distance between parallel lines of L1330 L1329
  measures "d285" distance of L1329.start L1324.start
  measures "d286" distance between parallel lines of L1333 L1321
  measures "d287" distance of L1325.start L1322.start
  measures "d288" distance of L1322.start L1322.end
  measures "d289" distance of L1340.end L1342.start
  measures "d290" distance of L1342.start L1339.start
  measures "d291" distance between parallel lines of L1328 L1341
  measures "d292" distance between parallel lines of L1343 L1320
  measures "d294" distance of L1354.end L1353.end
  measures "d295" distance of L1353.end L1352.end
extrude "Extrusion2" add sketch "Sketch10" along normal blind 1.5
body "Solid2"
